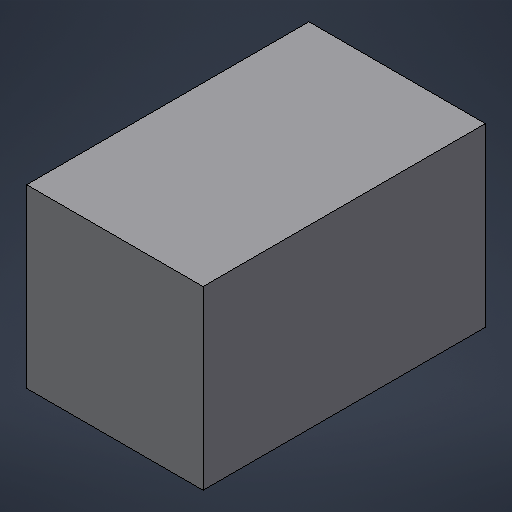
# Autodesk Inventor part: SampleQuader
Saved by Autodesk Inventor 2026.2 (Build 302298000, 298)
## iProperties
Created: 2026-03-26
Part Number: SampleQuader
Material: Generisch
Document SubType Name: Modeling
Designer: twiesendanger
Density: 1 g/cm^3
Appearance: Vorgabe
Author: twiesendanger
Autodesk Inventor part; units mm, degrees
ref_plane "YZ Plane" through (0, 0, 0) normal (1, 0, 0) x (0, 1, 0)
ref_plane "XZ Plane" through (0, 0, 0) normal (0, 1, 0) x (-1, 0, 0)
ref_plane "XY Plane" through (0, 0, 0) normal (0, 0, 1) x (1, 0, 0)
sketch "Sketch1" plane through (0, 0, 0) normal (0, 1, 0) x (-1, 0, 0)
  line L0 (25, -40) -> (-25, -40)
  line L1 (-25, -40) -> (-25, 40)
  line L2 (-25, 40) -> (25, 40)
  line L3 (25, 40) -> (25, -40)
  line L4 (25, -40) -> (-25, 40) construction
  line L5 (-25, -40) -> (25, 40) construction
  point P0 (0, 0)
  dimension "d0" = 50
  dimension "d1" = 80
  constraints: 12 end point, 2 midpoint, 2 parallel, 1 horizontal, 1 perpendicular
  measures "d0" distance of L1.end L2.end
  measures "d1" distance of L0.end L1.end
extrude "Extrusion1" add sketch "Sketch1" along normal blind 50
body "Solid1"
